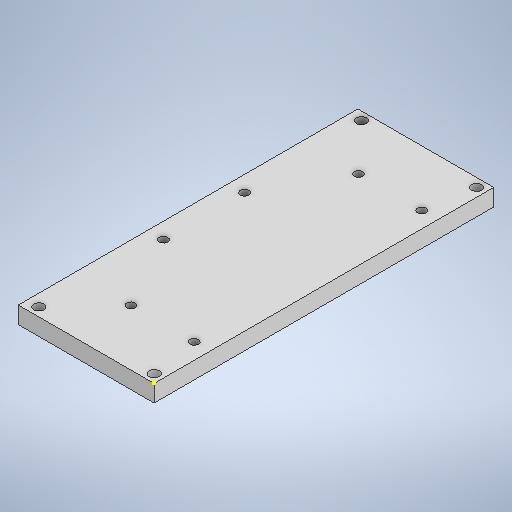
# Autodesk Inventor part: Base
Saved by Autodesk Inventor 2025.2 (Build 292293000, 293)
## iProperties
Created: 2025-01-27
Part Number: Base
Material: Genérico
Document SubType Name: Modeling
Designer: alex
Density: 1 g/cm^3
Appearance: Valor por defecto
Author: alex
Autodesk Inventor part; units mm, degrees
ref_plane "YZ Plane" through (0, 0, 0) normal (1, 0, 0) x (0, 1, 0)
ref_plane "XZ Plane" through (0, 0, 0) normal (0, 1, 0) x (-1, 0, 0)
ref_plane "XY Plane" through (0, 0, 0) normal (0, 0, 1) x (1, 0, 0)
sketch "Boceto1" plane through (0, 0, 0) normal (0, 1, 0) x (-1, 0, 0)
  line L0 (0, 0) -> (40, 0)
  line L1 (40, 0) -> (40, -100)
  line L2 (40, -100) -> (0, -100)
  line L3 (0, -100) -> (0, 0)
  circle A0 centre (19.95, -16.5) radius 1.5
  circle A1 centre (4, -16.5) radius 1.5
  circle A2 centre (19.95, -83.5) radius 1.5
  circle A3 centre (4, -83.5) radius 1.5
  point P0 (20, 0)
  dimension "d0" = 40
  dimension "d1" = 100
  dimension "d2" = 3
  dimension "d3" = 3
  dimension "d4" = 3
  dimension "d5" = 3
  dimension "d6" = 16.5
  dimension "d7" = 4
  dimension "d8" = 15.95
  dimension "d9" = 16.5
  dimension "d10" = 16.5
  dimension "d11" = 16.5
  dimension "d12" = 4
  dimension "d13" = 15.95
  constraints: 8 end point, 4 centre point, 2 parallel, 1 horizontal, 1 midpoint, 1 perpendicular
  measures "d0" distance of L1.end L2.end
  measures "d1" distance of L0.end L1.end
  measures "d2" diameter of A0
  measures "d3" diameter of A1
  measures "d4" diameter of A2
  measures "d5" diameter of A3
  measures "d6" distance from line of L0 A1.centre
  measures "d7" distance from line of L3 A1.centre
  measures "d8" distance of A0.centre A1.centre
  measures "d9" vertical distance of point (20, 0) A0.centre
  measures "d10" distance from line of L2 A2.centre
  measures "d11" distance from line of L2 A3.centre
  measures "d12" distance from line of L3 A3.centre
  measures "d13" distance of A3.centre A2.centre
extrude "Extrusión1" add sketch "Boceto1" along normal blind 5
sketch "Boceto2" plane through (0, 5, 0) normal (0, 1, 0) x (1, 0, 0)
  circle A0 centre (-2.5, 2.5) radius 1.5
  line L0 (0, 0) -> (0, 100) projected
  line L1 (-40, 0) -> (0, 0) projected
  circle A1 centre (-2.5, 97.5) radius 1.5
  line L2 (0, 100) -> (-40, 100) projected
  dimension "d16" = 3
  dimension "d17" = 2.5
  dimension "d18" = 2.5
  dimension "d19" = 3
  dimension "d20" = 2.5
  dimension "d21" = 2.5
  constraints: 2 centre point
  measures "d16" diameter of A0
  measures "d17" distance from line of L0 A0.centre
  measures "d18" distance from line of L1 A0.centre
  measures "d19" diameter of A1
  measures "d20" distance from line of L0 A1.centre
  measures "d21" distance from line of L2 A1.centre
extrude "Extrusión2" cut sketch "Boceto2" against normal blind 5
sketch "Boceto3" plane through (0, 5, 0) normal (0, 1, 0) x (1, 0, 0)
  line L0 (-40, 0) -> (0, 0) projected
  line L1 (-14.618, 24) -> (-8, 24)
  line L2 (-8, 24) -> (-8, 9)
  line L3 (-8, 9) -> (-14.618, 9)
  line L4 (-14.618, 9) -> (-14.618, 24)
  line L5 (0, 0) -> (0, 100) projected
  line L6 (-14.618, 91) -> (-8, 91)
  line L7 (-8, 91) -> (-8, 76)
  line L8 (-8, 76) -> (-14.618, 76)
  line L9 (-14.618, 76) -> (-14.618, 91)
  line L10 (0, 100) -> (-40, 100) projected
  dimension "d33" = 15
  dimension "d34" = 6.618
  dimension "d35" = 9
  dimension "d36" = 8
  dimension "d37" = 15
  dimension "d38" = 6.618
  dimension "d39" = 8
  dimension "d40" = 9
  constraints: 16 end point, 4 parallel, 2 horizontal, 2 perpendicular
  measures "d33" distance of L3.end L1.start
  measures "d34" distance between parallel lines of L2 L4
  measures "d35" distance between parallel lines of L0 L3
  measures "d36" distance between parallel lines of L5 L2
  measures "d37" distance of L6.end L7.end
  measures "d38" distance of L7.end L8.end
  measures "d39" distance between parallel lines of L5 L7
  measures "d40" distance between parallel lines of L10 L6
sketch "Boceto4" plane through (0, 5, 0) normal (0, 1, 0) x (1, 0, 0)
  point P0 (0, 0)
extrude "Extrusión3" cut sketch "Boceto3" against normal blind 0.5
sketch "Boceto5" plane through (0, 5, 0) normal (0, 1, 0) x (1, 0, 0)
  circle A0 centre (-19.95, 16.5) radius 1.5 projected
  circle A1 centre (-19.95, 16.5) radius 1.5
  circle A2 centre (-4, 16.5) radius 1.5 projected
  circle A3 centre (-4, 16.5) radius 1.5
  circle A4 centre (-19.95, 83.5) radius 1.5 projected
  circle A5 centre (-19.95, 83.5) radius 1.5
  circle A6 centre (-4, 83.5) radius 1.5 projected
  circle A7 centre (-4, 83.5) radius 1.5
  point P0 (0, 0)
  constraints: 4 centre point, 4 coincident
extrude "Extrusión4" add sketch "Boceto5" against normal blind 5
sketch "Boceto6" plane through (0, 5, 0) normal (0, 1, 0) x (1, 0, 0)
  line L0 (-8, 24) -> (-8, 9) projected
  line L1 (-8, 9) -> (-8, 16.5)
  line L2 (-8, 16.5) -> (-8, 19.5)
  line L3 (-14.618, 9) -> (-14.618, 24) projected
  line L4 (-14.618, 9) -> (-14.618, 16.5)
  circle A0 centre (-4, 16.5) radius 1.25
  circle A1 centre (-18.618, 16.5) radius 1.25
  circle A2 centre (-4, 83.5) radius 1.25
  circle A3 centre (-18.618, 83.5) radius 1.25
  line L5 (-8, 91) -> (-8, 76) projected
  line L6 (-14.618, 76) -> (-14.618, 91) projected
  line L7 (-14.618, 91) -> (-8, 91) projected
  point P0 (0, 0)
  dimension "d45" = 7.5
  dimension "d49" = 2.5
  dimension "d50" = 2.5
  dimension "d51" = 4
  dimension "d52" = 4
  dimension "d53" = 2.5
  dimension "d54" = 2.5
  dimension "d55" = 4
  dimension "d56" = 4
  dimension "d57" = 7.5
  dimension "d58" = 7.5
  constraints: 6 end point, 4 centre point, 4 midpoint, 1 point on line
  measures "d45" distance of L0.end L1.end
  measures "d49" diameter of A0
  measures "d50" diameter of A1
  measures "d51" distance of point (-8, 16.5) A0.centre
  measures "d52" distance of A1.centre point (-14.618, 16.5)
  measures "d53" diameter of A2
  measures "d54" diameter of A3
  measures "d55" distance from line of L5 A2.centre
  measures "d56" distance from line of L6 A3.centre
  measures "d57" distance from line of L7 A3.centre
  measures "d58" distance from line of L7 A2.centre
extrude "Extrusión5" cut sketch "Boceto6" against normal blind 5
sketch "Boceto7" plane through (0, 5, 0) normal (0, 1, 0) x (1, 0, 0)
  circle A0 centre (-18.618, 16.5) radius 1.25 projected
  circle A1 centre (-18.618, 16.5) radius 1.25
  circle A2 centre (-4, 16.5) radius 1.25 projected
  circle A3 centre (-4, 16.5) radius 1.25
  circle A4 centre (-18.618, 83.5) radius 1.25 projected
  circle A5 centre (-18.618, 83.5) radius 1.25
  circle A6 centre (-4, 83.5) radius 1.25 projected
  circle A7 centre (-4, 83.5) radius 1.25
  point P0 (0, 0)
  constraints: 4 centre point, 4 coincident
extrude "Extrusión6" add sketch "Boceto7" against normal blind 5
sketch "Boceto8" plane through (0, 5, 0) normal (0, 1, 0) x (1, 0, 0)
  circle A0 centre (-20.618, 16.5) radius 1.25
  circle A1 centre (-2, 16.5) radius 1.25
  line L0 (-8, 24) -> (-8, 9) projected
  line L1 (-14.618, 9) -> (-14.618, 24) projected
  line L2 (-8, 9) -> (-14.618, 9) projected
  circle A2 centre (-2, 83.5) radius 1.25
  circle A3 centre (-20.618, 83.5) radius 1.25
  line L3 (-14.618, 91) -> (-8, 91) projected
  line L4 (-8, 91) -> (-8, 76) projected
  line L5 (-14.618, 76) -> (-14.618, 91) projected
  point P0 (0, 0)
  point P1 (-8, 83.5)
  dimension "d63" = 2.5
  dimension "d64" = 2.5
  dimension "d65" = 6
  dimension "d66" = 6
  dimension "d67" = 7.5
  dimension "d68" = 7.5
  dimension "d69" = 2.5
  dimension "d70" = 2.5
  dimension "d71" = 7.5
  dimension "d72" = 7.5
  dimension "d73" = 6
  dimension "d74" = 6
  constraints: 4 centre point, 1 midpoint
  measures "d63" diameter of A0
  measures "d64" diameter of A1
  measures "d65" distance from line of A1.centre L0
  measures "d66" distance from line of L1 A0.centre
  measures "d67" distance from line of L2 A0.centre
  measures "d68" distance from line of L2 A1.centre
  measures "d69" diameter of A2
  measures "d70" diameter of A3
  measures "d71" distance from line of A3.centre L3
  measures "d72" distance from line of L3 A2.centre
  measures "d73" distance of point (-8, 83.5) A2.centre
  measures "d74" distance from line of L5 A3.centre
extrude "Extrusión7" cut sketch "Boceto8" against normal blind 6
sketch "Boceto9" plane through (0, 5, 0) normal (0, 1, 0) x (1, 0, 0)
  line L0 (-14.618, 9) -> (-14.618, 24) projected
  line L1 (-8, 24) -> (-8, 9) projected
  line L2 (-14.618, 24) -> (-8, 24)
  line L3 (-8, 24) -> (-8, 9)
  line L4 (-8, 9) -> (-14.618, 9)
  line L5 (-14.618, 9) -> (-14.618, 24)
  line L6 (-14.618, 91) -> (-8, 91) projected
  line L7 (-8, 76) -> (-14.618, 76) projected
  line L8 (-14.618, 91) -> (-8, 91)
  line L9 (-8, 91) -> (-8, 76)
  line L10 (-8, 76) -> (-14.618, 76)
  line L11 (-14.618, 76) -> (-14.618, 91)
  line L12 (-8, 91) -> (-8, 76) projected
  line L13 (-14.618, 91) -> (-8, 91)
  line L14 (-8, 91) -> (-8, 76)
  line L15 (-8, 76) -> (-14.618, 76)
  line L16 (-14.618, 76) -> (-14.618, 91)
  line L17 (-14.618, 24) -> (-8, 24)
  line L18 (-8, 24) -> (-8, 9)
  line L19 (-8, 9) -> (-14.618, 9)
  line L20 (-14.618, 9) -> (-14.618, 24)
  point P0 (0, 0)
  constraints: 32 end point, 8 parallel, 4 horizontal, 4 perpendicular
extrude "Extrusión8" add sketch "Boceto9" against normal blind 0.5
sketch "Boceto10" plane through (0, 5, 0) normal (0, 1, 0) x (1, 0, 0)
  circle A0 centre (-2, 16.5) radius 1.25 projected
  circle A1 centre (-2, 16.5) radius 1.25
  circle A2 centre (-4.691, 16.5) radius 1.25
  circle A3 centre (-23.309, 16.5) radius 1.25
  circle A4 centre (-20.618, 16.5) radius 1.25 projected
  circle A5 centre (-4.691, 83.5) radius 1.25
  circle A6 centre (-23.309, 83.5) radius 1.25
  circle A7 centre (-2, 83.5) radius 1.25 projected
  circle A8 centre (-20.618, 83.5) radius 1.25 projected
  point P0 (0, 0)
  dimension "d79" = 2.5
  dimension "d80" = 2.691
  dimension "d81" = 2.5
  dimension "d82" = 2.691
  dimension "d83" = 2.5
  dimension "d84" = 2.5
  dimension "d85" = 2.691
  dimension "d86" = 2.691
  constraints: 5 centre point, 1 coincident
  measures "d79" diameter of A2
  measures "d80" distance of A1.centre A2.centre
  measures "d81" diameter of A3
  measures "d82" distance of A4.centre A3.centre
  measures "d83" diameter of A5
  measures "d84" diameter of A6
  measures "d85" distance of A7.centre A5.centre
  measures "d86" distance of A6.centre A8.centre
extrude "Extrusión9" cut sketch "Boceto10" against normal blind 5 contours A2 | A3 | A5 | A6
sketch "Boceto11" plane through (0, 5, 0) normal (0, 1, 0) x (1, 0, 0)
  circle A0 centre (-20.618, 16.5) radius 1.25 projected
  circle A1 centre (-20.618, 16.5) radius 1.25
  circle A2 centre (-2, 16.5) radius 1.25 projected
  circle A3 centre (-2, 16.5) radius 1.25
  circle A4 centre (-20.618, 83.5) radius 1.25 projected
  circle A5 centre (-20.618, 83.5) radius 1.25
  circle A6 centre (-2, 83.5) radius 1.25 projected
  circle A7 centre (-2, 83.5) radius 1.25
  point P0 (0, 0)
  constraints: 4 centre point, 4 coincident
extrude "Extrusión10" add sketch "Boceto11" against normal blind 5
sketch "Boceto12" plane through (0, 5, 0) normal (0, 1, 0) x (1, 0, 0)
  circle A0 centre (-36.5, 2.5) radius 1.5
  circle A1 centre (-2.5, 2.5) radius 1.5 projected
  circle A2 centre (-36.5, 97.5) radius 1.5
  circle A3 centre (-2.5, 97.5) radius 1.5 projected
  point P0 (0, 0)
  dimension "d91" = 3
  dimension "d92" = 34
  dimension "d93" = 3
  dimension "d94" = 34
  constraints: 2 centre point
  measures "d91" diameter of A0
  measures "d92" distance of A0.centre A1.centre
  measures "d93" diameter of A2
  measures "d94" distance of A3.centre A2.centre
extrude "Extrusión11" cut sketch "Boceto12" against normal blind 10 contours A0 | A2
sketch "Boceto13" plane through (0, 5, 0) normal (0, 1, 0) x (1, 0, 0)
  circle A0 centre (-35.31, 38.04) radius 1.25
  circle A1 centre (-35.32, 61.96) radius 1.25
  line L0 (-40, 100) -> (-40, 0) projected
  line L1 (-40, 0) -> (0, 0) projected
  dimension "d97" = 2.5
  dimension "d98" = 2.5
  dimension "d99" = 23.92
  dimension "d100" = 4.68
  dimension "d101" = 4.69
  dimension "d102" = 38.04
  constraints: 2 centre point
  measures "d97" diameter of A0
  measures "d98" diameter of A1
  measures "d99" distance of A1.centre A0.centre
  measures "d100" distance from line of L0 A1.centre
  measures "d101" distance from line of L0 A0.centre
  measures "d102" distance from line of L1 A0.centre
extrude "Extrusión12" cut sketch "Boceto13" against normal blind 10
equation "\"d75\" = d73"
